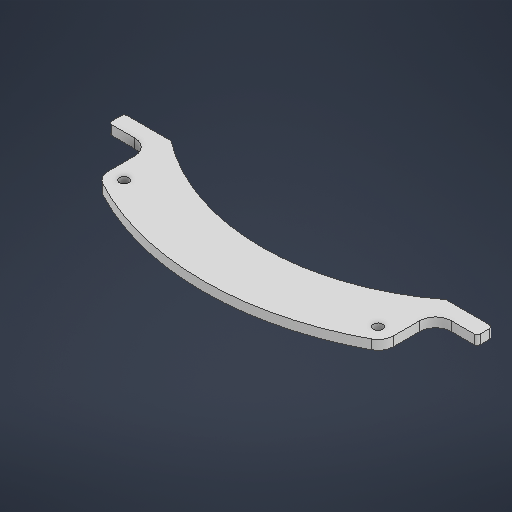
# Autodesk Inventor part: Parte B bastantes piezas
Saved by Autodesk Inventor 2026.2 (Build 302298000, 298)
## iProperties
Created: 2026-02-26
Part Number: Parte B bastantes piezas
Material: Generic
Document SubType Name: Modeling
Designer: 06aar
Density: 1 g/cm^3
Appearance: Default
Author: 06aar
Autodesk Inventor part; units mm, degrees
ref_plane "YZ Plane" through (0, 0, 0) normal (1, 0, 0) x (0, 1, 0)
ref_plane "XZ Plane" through (0, 0, 0) normal (0, 1, 0) x (-1, 0, 0)
ref_plane "XY Plane" through (0, 0, 0) normal (0, 0, 1) x (1, 0, 0)
sketch "Sketch1" plane through (0, 0, 0) normal (0, 1, 0) x (-1, 0, 0)
  circle A0 centre (0, 0) radius 75
  line L0 (0, 0) -> (45.6571, 59.5015)
  line L1 (0, 0) -> (-45.6571, 59.5015)
  line L2 (0, 0) -> (0, 75)
  circle A1 centre (0, 0) radius 72.3
  line L3 (44.0135, 57.3594) -> (59.0135, 57.3594)
  line L4 (-44.0135, 57.3594) -> (-59.0135, 57.3594)
  circle A2 centre (0, 0) radius 91
  line L5 (45.6571, 59.5015) -> (45.6571, 78.7174)
  line L6 (-45.6571, 59.5015) -> (-45.6571, 78.7174)
  line L7 (59.0135, 62.3594) -> (59.0135, 57.3594)
  line L8 (-59.0135, 62.3594) -> (-59.0135, 57.3594)
  line L9 (-45.6571, 62.3594) -> (-59.0135, 62.3594)
  line L10 (45.6571, 62.3594) -> (59.0135, 62.3594)
  dimension "d0" = 150
  dimension "d1" = 37.5
  dimension "d2" = 37.5
  dimension "d3" = 2.7
  dimension "d6" = 15
  dimension "d7" = 15
  dimension "d9" = 16
  dimension "d12" = 5
  dimension "d13" = 5
  constraints: 22 end point, 7 point on circle, 4 point on line, 3 centre point, 3 coincident, 3 horizontal, 3 parallel, 3 vertical, 1 concentric, 1 perpendicular
  measures "d0" diameter of A0
  measures "d1" angle of L1 L2
  measures "d2" angle of L2 L0
  measures "d3" radial gap between concentric circles of A0 A1
  measures "d6" distance of L4.start L4.end
  measures "d7" distance of L3.start L3.end
  measures "d9" radial gap between concentric circles of A2 A0
  measures "d12" distance between parallel lines of L4 L9
  measures "d13" distance of L7.start L3.end
extrude "Extrusion1" add sketch "Sketch1" along normal blind 3 contours L0 A1 L2 A0 | L5 L10 L7 L3 A0 | A0 L3 L0 | A0 L6 A2 L5 | L2 A1 L1 A0 | L1 L4 A0 | A0 L4 L8 L9 L6
fillet "Fillet1" radius 5 1 edges at (-45.6571, 1.5, 62.3594)
fillet "Fillet2" radius 5 3 edges at (45.6571, 1.5, 62.3594) (45.6571, 1.5, 78.7174) (-45.6571, 1.5, 78.7174)
fillet "Fillet3" radius 1 6 edges at (-44.0135, 1.5, 57.3594) (44.0135, 1.5, 57.3594) (59.0135, 1.5, 62.3594) (59.0135, 1.5, 57.3594) (-59.0135, 1.5, 57.3594) (-59.0135, 1.5, 62.3594)
sketch "Sketch2" plane through (0, 3, 0) normal (0, 1, 0) x (1, 0, 0)
  circle A0 centre (-40.6571, -75.7826) radius 1.5
  circle A1 centre (40.6571, -75.7826) radius 1.5
  arc A2 (-45.6571, -75.7826) -> (-43.0209, -80.1885) centre (-40.6571, -75.7826) ccw projected
  arc A3 (43.0209, -80.1885) -> (45.6571, -75.7826) centre (40.6571, -75.7826) ccw projected
  point P0 (0, 0)
  dimension "d17" = 3
  dimension "d18" = 3
  constraints: 2 centre point, 2 concentric
  measures "d17" diameter of A0
  measures "d18" diameter of A1
extrude "Extrusion2" cut sketch "Sketch2" against normal blind 3
body "Solid1"
